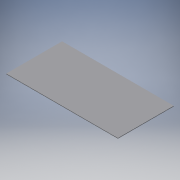
# Autodesk Inventor part: Pared ESTE Y OESTE
Saved by Autodesk Inventor 2016 (Build 200138000, 138)
## iProperties
Created: 2015-11-12
Part Number: Pared ESTE Y OESTE
Material: Generic
Document SubType Name: Modeling
Designer: serge
Density: 1 g/cm^3
Mass: 2.54e+06 g
Surface Area: 1.01524e+06 cm^2
Volume: 2.54e+06 cm^3
Appearance: Valor por defecto
Author: serge
Autodesk Inventor part; units mm, degrees
ref_plane "YZ Plane" through (0, 0, 0) normal (1, 0, 0) x (0, 1, 0)
ref_plane "XZ Plane" through (0, 0, 0) normal (0, 1, 0) x (-1, 0, 0)
ref_plane "XY Plane" through (0, 0, 0) normal (0, 0, 1) x (1, 0, 0)
sketch "Sketch1" plane through (0, 0, 0) normal (0, 0, 1) x (1, 0, 0)
  line L0 (-3503.0478, 11.274) -> (-3.0478, 11.274)
  line L1 (-3.0478, 11.274) -> (-3.0478, -3488.726)
  line L2 (-3.0478, -3488.726) -> (-3503.0478, -3488.726)
  line L3 (-3503.0478, -3488.726) -> (-3503.0478, 11.274)
  line L4 (-3503.0478, 11.274) -> (-3.0478, -3488.726) construction
  line L5 (-3.0478, 11.274) -> (-3503.0478, -3488.726) construction
  point P0 (0, 0)
  point P1 (-1753.0478, -1738.726)
  dimension "Largo" = 3500
  dimension "Alto" = 3500
  constraints: 12 end point, 2 midpoint, 2 parallel, 1 horizontal, 1 perpendicular
  measures "Largo" distance of L0.start L0.end
  measures "Alto" distance of L0.end L1.end
extrude "Extrusion1" add sketch "Sketch1" along normal blind 101.6
equation "\"Largo\" = PL_EO"
equation "\"Alto\" = PA_EO"
equation "\"Espesor\" = PE_EO"
equation "\"PL_EO\" = 3500"
equation "\"PA_EO\" = 3500"
equation "\"PE_EO\" = 101.6"
equation "\"PE_N\" = 101.6"
equation "\"PE_S\" = 101.6"
equation "\"T_E\" = 101.6"
equation "\"lon_ve\" = 512.5"
equation "\"n_a\" = 3"
equation "\"t_a\" = 19.05"
equation "\"d_a\" = 128.125"
equation "\"lon_ho\" = 749"
equation "\"d_bor\" = 59.92"
equation "\"lon_gui\" = 187.25"
equation "\"esp_gui\" = 461.25"
equation "\"lon_ve2\" = 498.475"
equation "\"n_a2\" = 3"
equation "\"t_a2\" = 124.61875"
equation "\"d_a2\" = 124.61875"
equation "\"lon_ho2\" = 933.45"
equation "\"d_bor2\" = 74.676"
equation "\"lon_gui2\" = 233.3625"
equation "\"esp_gui2\" = 448.6275"
equation "\"UE_L\" = 2671"
equation "\"UE_A\" = 1025"
equation "\"UE_AN\" = 749"
equation "\"UC_L\" = 1314.45"
equation "\"UC_A\" = 996.95"
equation "\"UC_AN\" = 933.45"
equation "\"A_ET\" = 35"
equation "\"SEP_NS\" = 0"
equation "\"DSEG\" = 0"
equation "\"AEGEP_NS\" = 0"
equation "\"DNS\" = 749"
body "Solid1"
